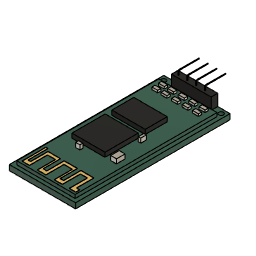
三维模型 v7 (Autodesk Fusion 360 archive; units mm, degrees)
design "无标题"
Autodesk Fusion 360 part; units mm, degrees
sketch "草图1" plane through (0, 0, 0) normal (0, 0, 1) x (1, 0, 0)
  line L0 (20, 35) -> (35, 35)
  line L1 (35, 35) -> (35, 0.0178)
  line L2 (35, 0.0178) -> (20, 0.0178)
  line L3 (20, 0.0178) -> (20, 35)
  dimension "d2" = 15
  constraint horizontal L0
  constraint vertical L1
  constraint horizontal L2
  constraint vertical L3
  measures "d2" distance of L0.start L0.end
extrude "拉伸1" add sketch "草图1" along normal blind 2 makes body 1
sketch "草图2" plane through (0, 0, 2) normal (0, 0, 1) x (-1, 0, 0)
  line L0 (-20, -0.0178) -> (-35, -0.0178)
  line L1 (-35, -0.0178) -> (-35, -35)
  line L2 (-35, -35) -> (-20, -35)
  line L3 (-20, -35) -> (-20, -0.0178)
  line L4 (-22.5, -11.4695) -> (-30, -11.4695)
  line L5 (-30, -11.4695) -> (-30, -19)
  line L6 (-30, -19) -> (-22.5, -19)
  line L7 (-22.5, -19) -> (-22.5, -11.4695)
  line L8 (-22.5, -20.5) -> (-30.07, -20.5)
  line L9 (-30.07, -20.5) -> (-30.07, -25.4841)
  line L10 (-30.07, -25.4841) -> (-22.5, -25.4841)
  line L11 (-22.5, -25.4841) -> (-22.5, -20.5)
  line L12 (-23, -35) -> (-23, -33.515)
  line L13 (-23, -33.515) -> (-32, -33.515)
  line L14 (-32, -33.515) -> (-32, -35)
  line L15 (-23, -35) -> (-32, -35)
  line L16 (-32, -33.515) -> (-23, -33.515)
  circle A0 centre (-21, -34) radius 0.5242
  circle A1 centre (-34, -34) radius 0.5259
  line L17 (-20.895, -33) -> (-34, -33)
  line L18 (-34, -33) -> (-34, -1)
  line L19 (-34, -1) -> (-20.895, -1)
  line L20 (-20.895, -1) -> (-20.895, -33)
  line L21 (-30.6999, -19.5528) -> (-31.2773, -19.5528)
  line L22 (-31.2773, -19.5528) -> (-31.2773, -18.2931)
  line L23 (-31.2773, -18.2931) -> (-30.6999, -18.2931)
  line L24 (-30.6999, -18.2931) -> (-30.6999, -19.5528)
  line L25 (-31.2773, -13.4116) -> (-32.5895, -13.4116)
  line L26 (-32.5895, -13.4116) -> (-32.5895, -11.4695)
  line L27 (-32.5895, -11.4695) -> (-31.2773, -11.4695)
  line L28 (-31.2773, -11.4695) -> (-31.2773, -13.4116)
  line L29 (-24.729, -10.7511) -> (-25.7263, -10.7511)
  line L30 (-25.7263, -10.7511) -> (-25.7263, -10.0688)
  line L31 (-25.7263, -10.0688) -> (-24.729, -10.0688)
  line L32 (-24.729, -10.0688) -> (-24.729, -10.7511)
  line L33 (-21.3696, -5.8171) -> (-21.3696, -1.3031)
  line L34 (-21.3696, -1.3031) -> (-23.0493, -1.3031)
  line L35 (-23.0493, -1.3031) -> (-23.0493, -5.3972)
  line L36 (-23.0493, -5.3972) -> (-24.8339, -5.3972)
  line L37 (-24.8339, -5.3972) -> (-24.8339, -1.3031)
  line L38 (-24.8339, -1.3031) -> (-26.776, -1.3031)
  line L39 (-26.776, -1.3031) -> (-26.776, -5.3972)
  line L40 (-26.776, -5.3972) -> (-28.6657, -5.3972)
  line L41 (-28.6657, -5.3972) -> (-28.6657, -1.3031)
  line L42 (-28.6657, -1.3031) -> (-30.5028, -1.3031)
  line L43 (-30.5028, -1.3031) -> (-30.5028, -5.3972)
  line L44 (-30.5028, -5.3972) -> (-32.0775, -5.3972)
  line L45 (-32.0775, -5.3972) -> (-32.0775, -1.3031)
  line L46 (-32.0775, -1.3031) -> (-33.5472, -1.3031)
  line L47 (-33.5472, -1.3031) -> (-33.5472, -2.1954)
  line L48 (-33.5472, -2.1954) -> (-32.8123, -2.1954)
  line L49 (-32.8123, -2.1954) -> (-32.8123, -6.1321)
  line L50 (-32.8123, -6.1321) -> (-29.8729, -6.1321)
  line L51 (-29.8729, -6.1321) -> (-29.8729, -2.1954)
  line L52 (-29.8729, -2.1954) -> (-29.0856, -2.1954)
  line L53 (-29.0856, -2.1954) -> (-29.0856, -6.1321)
  line L54 (-29.0856, -6.1321) -> (-26.0937, -6.1321)
  line L55 (-26.0937, -6.1321) -> (-26.0937, -2.1954)
  line L56 (-26.0937, -2.1954) -> (-25.2539, -2.1954)
  line L57 (-25.2539, -2.1954) -> (-25.2539, -6.1321)
  line L58 (-25.2539, -6.1321) -> (-22.4194, -6.1321)
  line L59 (-22.4194, -6.1321) -> (-22.4194, -2.1954)
  line L60 (-22.4194, -2.1954) -> (-21.8421, -2.1954)
  line L61 (-21.8421, -2.1954) -> (-21.8421, -6.7094)
  line L62 (-21.8421, -6.7094) -> (-21.3172, -6.7094)
  line L63 (-21.3172, -6.7094) -> (-21.3696, -5.8171)
  dimension "d6" = 1.5
  constraint horizontal L4
  constraint vertical L5
  constraint horizontal L6
  constraint vertical L7
  constraint horizontal L8
  constraint vertical L9
  constraint horizontal L10
  constraint vertical L11
  constraint coincident L2 L14.end
  constraint coincident L2 L12.start
  constraint perpendicular L2 L12
  constraint perpendicular L12 L13
  constraint perpendicular L14 L15
  constraint horizontal L17
  constraint vertical L18
  constraint horizontal L19
  constraint vertical L20
  constraint horizontal L21
  constraint vertical L22
  constraint horizontal L23
  constraint vertical L24
  constraint horizontal L25
  constraint vertical L26
  constraint horizontal L27
  constraint vertical L28
  constraint horizontal L29
  constraint vertical L30
  constraint horizontal L31
  constraint vertical L32
  constraint perpendicular L4 L33
  constraint perpendicular L7 L34
  constraint perpendicular L4 L35
  constraint perpendicular L35 L36
  constraint perpendicular L36 L37
  constraint perpendicular L35 L38
  constraint perpendicular L36 L39
  constraint perpendicular L39 L40
  constraint perpendicular L40 L41
  constraint perpendicular L41 L42
  constraint perpendicular L40 L43
  constraint perpendicular L43 L44
  constraint perpendicular L44 L45
  constraint perpendicular L43 L46
  constraint perpendicular L44 L47
  constraint perpendicular L47 L48
  constraint perpendicular L48 L49
  constraint perpendicular L49 L50
  constraint perpendicular L50 L51
  constraint perpendicular L41 L52
  constraint perpendicular L52 L53
  constraint perpendicular L53 L54
  constraint perpendicular L54 L55
  constraint perpendicular L55 L56
  constraint perpendicular L36 L57
  constraint perpendicular L57 L58
  constraint perpendicular L58 L59
  constraint perpendicular L59 L60
  constraint perpendicular L60 L61
  constraint perpendicular L61 L62
  measures "d6" distance of L6.end L8.start
extrude "拉伸1'" add sketch "草图2" along normal blind 1 separate body contours L2 L12 L13 L14 L15 L16 | L4 L5 L6 L7 | L8 L9 L10 L11 | A0 | A1 | L21 L22 L23 L24 | L25 L26 L27 L28 | L29 L30 L31 L32 | L33 L34 L35 L36 L37 L38 L39 L40 L41 L42 L43 L44 L45 L46 L47 L48 L49 L50 L51 L52 L53 L54 L55 L56 L57 L58 L59 L60 L61 L62 L63 makes body 2 at (31.7147, 12.7642, 2) makes body 3 at (33.7147, 33.5582, 2.6667) makes body 4 at (26, 34.505, 2) makes body 5 at (31.2773, 19.1329, 2.3333) makes body 6 at (25.0614, 10.7511, 2.3333) makes body 7 at (27.5467, 23.8227, 2) makes body 8 at (21.366, 34.3753, 2.6667) makes body 9 at (27.5, 13.9797, 2) makes body 10 at (25.9012, 1.6005, 2) in component "Component'"
extrude "拉伸2" cut 2 faces at (20.833, 34.2892, 3) (34.1675, 33.9483, 3) along direction (0, 0, -1) blind 12 on bodies 3 8 bodies 1
extrude "拉伸2'" cut 2 faces at (20.833, 34.2892, 3) (34.1675, 33.9483, 3) along direction (0, 0, -1) blind 12 on bodies 3 8 bodies 3 8 in component "Component'"
sketch "草图3" plane through (0, 0, 2) normal (0, 0, 1) x (-1, 0, 0)
  circle A0 centre (-21, -34) radius 0.5242
  circle A1 centre (-34, -34) radius 0.5259
  line L0 (-20, -0.0178) -> (-35, -0.0178)
  line L1 (-35, -0.0178) -> (-35, -35)
  line L2 (-35, -35) -> (-20, -35)
  line L3 (-20, -35) -> (-20, -0.0178)
  line L4 (-20.9214, -32.9294) -> (-34.1188, -32.9294)
  line L5 (-34.1188, -32.9294) -> (-34.1188, -0.8092)
  line L6 (-34.1188, -0.8092) -> (-20.9214, -0.8092)
  line L7 (-20.9214, -0.8092) -> (-20.9214, -32.9294)
  constraint horizontal L4
  constraint vertical L5
  constraint horizontal L6
  constraint vertical L7
extrude "拉伸3" cut sketch "草图3" against normal blind 0.8 bodies 1
extrude "拉伸3'" cut 1 faces at (25.9012, 1.6005, 3) along direction (0, 0, -1) blind 0.95 on bodies 10 bodies 10 in component "Component'"
move_body "移动1" bodies 1 to x (1, 0, 0) y (0, 1, 0) z (0, 0, 1) at (-1.5, 0, 0)
move_body "移动2" bodies 1 to x (1, 0, 0) y (0, 1, 0) z (0, 0, 1) at (-0.3, 0, 0)
extrude "拉伸4" add 1 faces at (26, 34.505, 2) along direction (0, 0, -1) blind 0.8 on bodies 4 bodies 4 3 8 in component "Component'"
move_body "移动3" bodies 1 to x (1, 0, 0) y (0, 1, 0) z (0, 0, 1) at (1.3, 0, 0)
move_body "移动4" bodies 1 to x (1, 0, 0) y (0, 1, 0) z (0, 0, 1) at (0.28, 0, 0)
extrude "拉伸5" add 1 faces at (26, 34.505, 3) along direction (0, 0, 1) blind 0.8 on bodies 4 bodies 4 in component "Component'"
sketch "草图4" plane through (0, 0, 0) normal (1, 0, 0) x (0, 1, 0)
  line L0 (33.9897, 3.8149) -> (33.9897, 4.8558)
  line L1 (33.9897, 4.8558) -> (38.7569, 4.8558)
  line L2 (38.7569, 4.8558) -> (38.7569, 4.6268)
  line L3 (38.7569, 4.6268) -> (34.2603, 4.6268)
  line L4 (34.2603, 4.6268) -> (34.2603, 3.8149)
  line L5 (34.2603, 3.8149) -> (33.9897, 3.8149)
  constraint vertical L0
  constraint perpendicular L0 L1
  constraint perpendicular L1 L2
  constraint perpendicular L2 L3
  constraint perpendicular L3 L4
  constraint perpendicular L0 L5
extrude "拉伸4'" add sketch "草图4" along normal blind 0.1 separate body makes body 11
fillet "圆角1" radius 0.2 1 edges at (0.05, 33.9897, 4.8558) on bodies 11
extrude "拉伸5'" cut 1 faces at (0.0333, 34.2603, 4.3561) along direction (0, -1, 0) blind 0.1 on bodies 11 bodies 11
extrude "拉伸6" cut 1 faces at (0.0333, 37.2247, 4.6268) along direction (0, 0, 1) blind 0.1 on bodies 11 bodies 11
fillet "圆角2" radius 0.2 1 edges at (0.05, 34.1603, 4.7268) on bodies 11
move_body "移动5" bodies 11 to x (1, 0, 0) y (0, 1, 0) z (0, 0, 1) at (24, 0, 0)
copy_body "复制和粘贴实体1" bodies 11 makes body 12
move_body "移动6" bodies 12 to x (1, 0, 0) y (0, 1, 0) z (0, 0, 1) at (2, 0, 0)
copy_body "复制和粘贴实体2" bodies 11 12 makes body 13 makes body 14
move_body "移动7" bodies 13 14 to x (1, 0, 0) y (0, 1, 0) z (0, 0, 1) at (4, 0, 0)
sketch "草图5" plane through (0, 0, 2) normal (0, 0, 1) x (-1, 0, 0)
  line L0 (-20.7014, -32.9294) -> (-20.7014, -0.8092)
  line L1 (-20.7014, -0.8092) -> (-33.8988, -0.8092)
  line L2 (-33.8988, -0.8092) -> (-33.8988, -32.9294)
  line L3 (-33.8988, -32.9294) -> (-20.7014, -32.9294)
  line L4 (-22.0123, -32.2902) -> (-23.3153, -32.2902)
  line L5 (-23.3153, -32.2902) -> (-23.3153, -31.5664)
  line L6 (-23.3153, -31.5664) -> (-22.0123, -31.5664)
  line L7 (-22.0123, -31.5664) -> (-22.0123, -32.2902)
  line L8 (-24.0874, -32.2902) -> (-25.4386, -32.2902)
  line L9 (-25.4386, -32.2902) -> (-25.4386, -31.5664)
  line L10 (-25.4386, -31.5664) -> (-24.0874, -31.5664)
  line L11 (-24.0874, -31.5664) -> (-24.0874, -32.2902)
  line L12 (-26.4645, -32.2902) -> (-27.847, -32.2902)
  line L13 (-27.847, -32.2902) -> (-27.847, -31.5664)
  line L14 (-27.847, -31.5664) -> (-26.4645, -31.5664)
  line L15 (-26.4645, -31.5664) -> (-26.4645, -32.2902)
  line L16 (-28.87, -32.2902) -> (-30.1972, -32.2902)
  line L17 (-30.1972, -32.2902) -> (-30.1972, -31.5664)
  line L18 (-30.1972, -31.5664) -> (-28.87, -31.5664)
  line L19 (-28.87, -31.5664) -> (-28.87, -32.2902)
  line L20 (-31.1926, -32.2902) -> (-32.5474, -32.2902)
  line L21 (-32.5474, -32.2902) -> (-32.5474, -31.5664)
  line L22 (-32.5474, -31.5664) -> (-31.1926, -31.5664)
  line L23 (-31.1926, -31.5664) -> (-31.1926, -32.2902)
  line L24 (-24.0874, -30.0664) -> (-24.0874, -30.7902)
  line L25 (-32.5474, -30.7902) -> (-32.5474, -30.0664)
  line L26 (-31.1926, -30.7902) -> (-32.5474, -30.7902)
  line L27 (-27.847, -30.0664) -> (-26.4645, -30.0664)
  line L28 (-25.4386, -30.7902) -> (-25.4386, -30.0664)
  line L29 (-30.1972, -30.0664) -> (-28.87, -30.0664)
  line L30 (-28.87, -30.7902) -> (-30.1972, -30.7902)
  line L31 (-32.5474, -30.0664) -> (-31.1926, -30.0664)
  line L32 (-30.1972, -30.7902) -> (-30.1972, -30.0664)
  line L33 (-22.0123, -30.7902) -> (-23.3153, -30.7902)
  line L34 (-23.3153, -30.0664) -> (-22.0123, -30.0664)
  line L35 (-28.87, -30.0664) -> (-28.87, -30.7902)
  line L36 (-23.3153, -30.7902) -> (-23.3153, -30.0664)
  line L37 (-22.0123, -30.0664) -> (-22.0123, -30.7902)
  line L38 (-27.847, -30.7902) -> (-27.847, -30.0664)
  line L39 (-24.0874, -30.7902) -> (-25.4386, -30.7902)
  line L40 (-26.4645, -30.7902) -> (-27.847, -30.7902)
  line L41 (-26.4645, -30.0664) -> (-26.4645, -30.7902)
  line L42 (-25.4386, -30.0664) -> (-24.0874, -30.0664)
  line L43 (-31.1926, -30.0664) -> (-31.1926, -30.7902)
  constraint horizontal L4
  constraint vertical L5
  constraint horizontal L6
  constraint vertical L7
  constraint horizontal L8
  constraint vertical L9
  constraint horizontal L10
  constraint vertical L11
  constraint horizontal L12
  constraint vertical L13
  constraint horizontal L14
  constraint vertical L15
  constraint horizontal L16
  constraint vertical L17
  constraint horizontal L18
  constraint vertical L19
  constraint horizontal L20
  constraint vertical L21
  constraint horizontal L22
  constraint vertical L23
  constraint horizontal L33
  constraint vertical L36
  constraint horizontal L34
  constraint vertical L37
  constraint horizontal L39
  constraint vertical L28
  constraint horizontal L42
  constraint vertical L24
  constraint horizontal L40
  constraint vertical L38
  constraint horizontal L27
  constraint vertical L41
  constraint horizontal L30
  constraint vertical L32
  constraint horizontal L29
  constraint vertical L35
  constraint horizontal L26
  constraint vertical L25
  constraint horizontal L31
  constraint vertical L43
extrude "拉伸7" add sketch "草图5" along normal blind 0.5 separate body contours L4 L5 L6 L7 | L8 L9 L10 L11 | L12 L13 L14 L15 | L16 L17 L18 L19 | L20 L21 L22 L23 | L24 L28 L39 L42 | L25 L26 L31 L43 | L27 L38 L40 L41 | L29 L30 L32 L35 | L33 L34 L36 L37 makes body 15 at (22.4467, 30.549, 2) makes body 16 at (22.4467, 31.8077, 2) makes body 17 at (29.3124, 31.8077, 2) makes body 18 at (24.5378, 31.8077, 2) makes body 19 at (26.9253, 30.549, 2) makes body 20 at (24.5378, 30.3077, 2) makes body 21 at (26.9253, 32.049, 2) makes body 22 at (31.6442, 31.8077, 2) makes body 23 at (29.7548, 30.3077, 2) makes body 24 at (31.6442, 30.3077, 2)
form "造型1" [no effect]
component "Component'" placed x (1, 0, 0) y (0, 1, 0) z (0, 0, 1) at (0, 0, 0)
